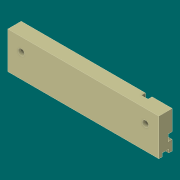
# Autodesk Inventor part: sensorHolder
Saved by Autodesk Inventor 2016 (Build 200138000, 138)
## iProperties
Created: 2015-10-19
Part Number: sensorHolder
Material: ABS Plastic
Document SubType Name: Modeling
Designer: Sawaiz
Density: 1.06 g/cm^3
Appearance: Smooth - Ash
Author: Sawaiz
Autodesk Inventor part; units mm, degrees
ref_plane "YZ Plane" through (0, 0, 0) normal (1, 0, 0) x (0, 1, 0)
ref_plane "XZ Plane" through (0, 0, 0) normal (0, 1, 0) x (-1, 0, 0)
ref_plane "XY Plane" through (0, 0, 0) normal (0, 0, 1) x (1, 0, 0)
sketch "Sketch1" plane through (0, 0, 0) normal (1, 0, 0) x (0, 1, 0)
  line L0 (-44.45, 44.45) -> (44.45, 44.45)
  line L1 (44.45, 44.45) -> (44.45, 0)
  line L2 (44.45, 0) -> (-44.45, 0)
  line L3 (-44.45, 0) -> (-44.45, 44.45)
  line L4 (-44.45, 44.45) -> (44.45, 0) construction
  line L5 (44.45, 44.45) -> (-44.45, 0) construction
  line L6 (-26.9875, 0) -> (26.9875, 0)
  line L7 (26.9875, 0) -> (26.9875, 26.9875)
  line L8 (26.9875, 26.9875) -> (-26.9875, 26.9875)
  line L9 (-26.9875, 26.9875) -> (-26.9875, 0)
  line L10 (-26.9875, 26.9875) -> (-26.9875, 44.45)
  line L11 (26.9875, 26.9875) -> (44.45, 26.9875)
  point P0 (0, 0)
  point P1 (0, 22.225)
  point P2 (0, 0)
  dimension "d5" = 88.9
  dimension "d6" = 44.45
  dimension "d7" = 53.975
  dimension "d8" = 26.9875
  constraints: 24 end point, 4 midpoint, 4 parallel, 3 horizontal, 3 point on line, 2 perpendicular, 1 coincident, 1 vertical
  measures "d5" distance between parallel lines of L3 L1
  measures "d6" distance of L0.end L1.end
  measures "d7" distance of L7.end L8.end
  measures "d8" distance of L6.end L7.end
extrude "Extrusion1" add sketch "Sketch1" along normal blind 6.35 contours L0 L1 L11 L8 L10
sketch "Sketch2" plane through (0, -26.9875, 26.9875) normal (0, 0, -1) x (-1, 0, 0)
  line L0 (0, 0) -> (0, 71.4375) projected
  line L1 (0, 71.4375) -> (-6.35, 71.4375) projected
  line L2 (-6.35, 0) -> (-6.35, 71.4375) projected
  line L3 (0, 0) -> (-6.35, 0) projected
  line L4 (-3.175, 0) -> (-3.175, 71.4375)
  line L5 (-4.7625, 0) -> (-1.5875, 0)
  line L6 (-1.5875, 0) -> (-1.5875, 71.4375)
  line L7 (-1.5875, 71.4375) -> (-4.7625, 71.4375)
  line L8 (-4.7625, 71.4375) -> (-4.7625, 0)
  line L9 (-4.7625, 0) -> (-1.5875, 71.4375) construction
  line L10 (-1.5875, 0) -> (-4.7625, 71.4375) construction
  point P0 (0, 26.9875)
  point P1 (-3.175, 35.7187)
  dimension "d11" = 3.175
  constraints: 14 end point, 5 midpoint, 2 parallel, 1 collinear, 1 horizontal, 1 perpendicular
  measures "d11" distance between parallel lines of L8 L6
extrude "Extrusion2" cut sketch "Sketch2" against normal blind 1.5875 contours L3 L4 L1 L6 | L3 L8 L1 L4
sketch "Sketch3" plane through (6.35, 0, 0) normal (1, 0, 0) x (0, 0, -1)
  line L0 (-26.9875, -26.9875) -> (-26.9875, 44.45) projected
  line L1 (-26.9875, 44.45) -> (-44.45, 44.45) projected
  line L2 (-44.45, 44.45) -> (-44.45, -26.9875) projected
  line L3 (-44.45, -26.9875) -> (-26.9875, -26.9875) projected
  line L4 (-38.1, -20.6375) -> (-38.1, 38.1)
  point P0 (0, 0)
  dimension "d14" = 6.35
  dimension "d15" = 6.35
  dimension "d16" = 6.35
  constraints: 2 end point, 1 vertical
  measures "d14" distance from line of L2 L4.start
  measures "d15" distance from line of L3 L4.start
  measures "d16" distance from line of L1 L4.end
hole "Hole1" at (6.35, -20.6375, 38.1) at (6.35, 38.1, 38.1) direction (-1, 0, 0) diameter 1.778 end through all countersink diameter 3.023 countersink angle 82 clearance for "Flat Head Machine Screw (82)" size "#0" standard "Ansi Unified Screw Threads"
sketch "Sketch4" plane through (0, 0, 0) normal (-1, 0, 0) x (0, 0, 1)
  line L0 (-31.75, -31.75) -> (31.75, -31.75)
  line L1 (31.75, -31.75) -> (31.75, 31.75)
  line L2 (31.75, 31.75) -> (-31.75, 31.75)
  line L3 (-31.75, 31.75) -> (-31.75, -31.75)
  line L4 (-31.75, -31.75) -> (31.75, 31.75) construction
  line L5 (31.75, -31.75) -> (-31.75, 31.75) construction
  line L6 (-34.925, 34.925) -> (34.925, 34.925)
  line L7 (34.925, 34.925) -> (34.925, -34.925)
  line L8 (34.925, -34.925) -> (-34.925, -34.925)
  line L9 (-34.925, -34.925) -> (-34.925, 34.925)
  line L10 (-34.925, 34.925) -> (34.925, -34.925) construction
  line L11 (34.925, 34.925) -> (-34.925, -34.925) construction
  line L12 (26.9875, 44.45) -> (44.45, 44.45) projected
  line L13 (31.75, 31.75) -> (34.925, 31.75)
  line L14 (34.925, 31.75) -> (34.925, 44.45)
  line L15 (34.925, 44.45) -> (31.75, 44.45)
  line L16 (31.75, 44.45) -> (31.75, 31.75)
  line L17 (31.75, 31.75) -> (44.45, 31.75)
  line L18 (44.45, 31.75) -> (44.45, 34.925)
  line L19 (44.45, 34.925) -> (31.75, 34.925)
  line L20 (31.75, 34.925) -> (31.75, 31.75)
  line L21 (44.45, 44.45) -> (44.45, -26.9875) projected
  point P0 (0, 0)
  dimension "d24" = 63.5
  dimension "d25" = 63.5
  dimension "d26" = 3.175
  dimension "d27" = 3.175
  constraints: 40 end point, 8 parallel, 4 horizontal, 4 midpoint, 4 perpendicular, 3 collinear, 1 point on line
  measures "d24" distance of L0.end L1.end
  measures "d25" distance between parallel lines of L3 L1
  measures "d26" distance between parallel lines of L1 L7
  measures "d27" distance between parallel lines of L2 L6
extrude "Extrusion3" cut sketch "Sketch4" against normal blind 1.905 contours L13 L7 L8 L9 L6 L16 | L16 L6 L7 L13 | L7 L19 L18 L17 | L16 L12 L14 L6
equation "\"d5\" = sensorHolderWidth"
equation "\"d6\" = 0.5 * sensorHolderHeight"
equation "\"d7\" = sensorHolderSensorWidth"
equation "\"d8\" = 0.5 * sensorHolderSesnorHeight"
equation "\"d9\" = acrylicThickness"
equation "\"d11\" = oRingWidth"
equation "\"d12\" = 0.5 * oRingWidth"
equation "\"d14\" = acrylicThickness"
equation "\"d15\" = acrylicThickness"
equation "\"d16\" = acrylicThickness"
equation "\"d24\" = 0.25 * sensorHolderFlushORingID"
equation "\"d25\" = 0.25 * sensorHolderFlushORingID"
equation "\"d26\" = oRingWidth"
equation "\"d27\" = oRingWidth"
equation "\"acrylicThickness\" = 6.35"
equation "\"height\" = 101.6"
equation "\"width\" = 101.6"
equation "\"depth\" = 101.6"
equation "\"mirrorAngle\" = 5deg"
equation "\"detectorWidth\" = 52"
equation "\"detectorHeight\" = 52"
equation "\"mirrorThickness\" = 3"
equation "\"fresnelThickness\" = 0.1"
equation "\"focalLength\" = 76.2"
equation "\"ior\" = 1.49"
equation "\"centerThickness\" = 1.524"
equation "\"fresnelAngle\" = 90deg"
equation "\"fresnelEffectiveDiameter\" = 76.2"
equation "\"mirrorSuppourtWidth\" = 38.1"
equation "\"backGrooveBit\" = 4.8006"
equation "\"sensorHolderWidth\" = 88.9"
equation "\"sensorHolderHeight\" = 88.9"
equation "\"sensorHolderSesnorHeight\" = 53.975"
equation "\"sensorHolderSensorWidth\" = 53.975"
equation "\"sensorHolderSensorHeight\" = 53.975"
equation "\"sensorHolderORingGroove\" = 3.175"
equation "\"sensorHolderORing\" = 3.175"
equation "\"sensorHolderFlushORing\" = 3.175"
equation "\"sensorHolderFlushORingID\" = 254"
equation "\"frontBackORingID\" = 419.1"
equation "\"oRingWidth\" = 3.175"
equation "\"sensorHolderORingID\" = 203.2"
equation "\"topBottomHorizontalMirrorGroove\" = 12.7"
equation "\"backMirrorGroove\" = 6.35"
equation "\"mirrorGroove\" = 19.05"
equation "\"fresnelChamfer\" = 6.35"
equation "\"mirrorGrooveFillet\" = 6.35"
equation "\"mirrorGrooveDrill\" = 6.35"
equation "\"mirrorGrooveMill\" = 3.175"
body "Solid1"
